Autodesk Fusion 360 part; units mm, degrees
(part 3 of 5)
sketch "草图7 (11)" plane through (0, 0, 0) normal (0, 0, 1) x (1, 0, 0) in component "RS_Integrated"
  line L0 (779, 145) -> (860, 145)
  line L1 (860, 145) -> (860, 153)
  line L2 (860, 153) -> (779, 153)
  line L3 (779, 153) -> (779, 145)
  dimension "d1107" = 779
  dimension "d1108" = 145
  dimension "d1109" = 81
  dimension "d1110" = 8
  constraint horizontal L0
  constraint vertical L1
  constraint horizontal L2
  constraint vertical L3
  measures "d1107" horizontal distance of origin L0.start
  measures "d1108" vertical distance of origin L0.start
  measures "d1109" horizontal distance of L0.start L0.end
  measures "d1110" vertical distance of L0.end L1.end
extrude "R05 low integral runner 0'''''" add sketch "草图7 (11)" along normal blind 10 bodies 11 in component "RS_Integrated"
ref_plane "工作平面8" through (0, 0, 0) normal (0, 0, 1) x (1, 0, 0) in component "RS_Integrated"
sketch "草图8 (11)" plane through (0, 0, 0) normal (0, 0, 1) x (1, 0, 0) in component "RS_Integrated"
  line L0 (779, 311) -> (860, 311)
  line L1 (860, 311) -> (860, 319)
  line L2 (860, 319) -> (779, 319)
  line L3 (779, 319) -> (779, 311)
  dimension "d1115" = 779
  dimension "d1116" = 311
  dimension "d1117" = 81
  dimension "d1118" = 8
  constraint horizontal L0
  constraint vertical L1
  constraint horizontal L2
  constraint vertical L3
  measures "d1115" horizontal distance of origin L0.start
  measures "d1116" vertical distance of origin L0.start
  measures "d1117" horizontal distance of L0.start L0.end
  measures "d1118" vertical distance of L0.end L1.end
extrude "R05 low integral runner 1'''''" add sketch "草图8 (11)" along normal blind 10 bodies 11 in component "RS_Integrated"
chamfer "倒角1''''''''''" distance 0.4 angle 45 5 edges at (813.5, 145, 35) (813.5, 319, 35) (857, 232, 35) (815, 142, 35) (815, 322, 35) on bodies 11 in component "RS_Integrated"
ref_plane "工作平面1" through (0, 0, 26) normal (0, 0, 1) x (1, 0, 0) in component "RS_RemovableGrate"
sketch "草图1 (12)" plane through (0, 0, 26) normal (0, 0, 1) x (1, 0, 0) in component "RS_RemovableGrate"
  line L0 (773.3, 145.3) -> (856.7, 145.3)
  line L1 (856.7, 145.3) -> (856.7, 318.7)
  line L2 (856.7, 318.7) -> (773.3, 318.7)
  line L3 (773.3, 318.7) -> (773.3, 145.3)
  dimension "d1124" = 773.3
  dimension "d1126" = 83.4
  dimension "d1127" = 173.4
  constraint horizontal L0
  constraint vertical L1
  constraint horizontal L2
  constraint vertical L3
  measures "d1124" horizontal distance of origin L0.start
  measures "d1126" horizontal distance of L0.start L0.end
  measures "d1127" vertical distance of L0.end L1.end
extrude "Horizontal removable deck'''''" add sketch "草图1 (12)" along normal blind 4 separate body makes body 12 in component "RS_RemovableGrate"
ref_plane "工作平面2" through (0, 0, 26) normal (0, 0, 1) x (1, 0, 0) in component "RS_RemovableGrate"
sketch "草图2 (12)" plane through (0, 0, 26) normal (0, 0, 1) x (1, 0, 0) in component "RS_RemovableGrate"
  line L0 (780.3, 160) -> (849.7, 160)
  line L1 (849.7, 160) -> (849.7, 164)
  line L2 (849.7, 164) -> (780.3, 164)
  line L3 (780.3, 164) -> (780.3, 160)
  dimension "d1132" = 780.3
  dimension "d1133" = 160
  dimension "d1134" = 69.4
  dimension "d1135" = 4
  constraint horizontal L0
  constraint vertical L1
  constraint horizontal L2
  constraint vertical L3
  measures "d1132" horizontal distance of origin L0.start
  measures "d1133" vertical distance of origin L0.start
  measures "d1134" horizontal distance of L0.start L0.end
  measures "d1135" vertical distance of L0.end L1.end
extrude "Drain slot 1'''''" cut sketch "草图2 (12)" along normal blind 4 bodies 12 in component "RS_RemovableGrate"
ref_plane "工作平面3" through (0, 0, 26) normal (0, 0, 1) x (1, 0, 0) in component "RS_RemovableGrate"
sketch "草图3 (12)" plane through (0, 0, 26) normal (0, 0, 1) x (1, 0, 0) in component "RS_RemovableGrate"
  line L0 (780.3, 170) -> (849.7, 170)
  line L1 (849.7, 170) -> (849.7, 174)
  line L2 (849.7, 174) -> (780.3, 174)
  line L3 (780.3, 174) -> (780.3, 170)
  dimension "d1140" = 780.3
  dimension "d1141" = 170
  dimension "d1142" = 69.4
  dimension "d1143" = 4
  constraint horizontal L0
  constraint vertical L1
  constraint horizontal L2
  constraint vertical L3
  measures "d1140" horizontal distance of origin L0.start
  measures "d1141" vertical distance of origin L0.start
  measures "d1142" horizontal distance of L0.start L0.end
  measures "d1143" vertical distance of L0.end L1.end
extrude "Drain slot 2'''''" cut sketch "草图3 (12)" along normal blind 4 bodies 12 in component "RS_RemovableGrate"
ref_plane "工作平面4" through (0, 0, 26) normal (0, 0, 1) x (1, 0, 0) in component "RS_RemovableGrate"
sketch "草图4 (12)" plane through (0, 0, 26) normal (0, 0, 1) x (1, 0, 0) in component "RS_RemovableGrate"
  line L0 (780.3, 180) -> (849.7, 180)
  line L1 (849.7, 180) -> (849.7, 184)
  line L2 (849.7, 184) -> (780.3, 184)
  line L3 (780.3, 184) -> (780.3, 180)
  dimension "d1148" = 780.3
  dimension "d1149" = 180
  dimension "d1150" = 69.4
  dimension "d1151" = 4
  constraint horizontal L0
  constraint vertical L1
  constraint horizontal L2
  constraint vertical L3
  measures "d1148" horizontal distance of origin L0.start
  measures "d1149" vertical distance of origin L0.start
  measures "d1150" horizontal distance of L0.start L0.end
  measures "d1151" vertical distance of L0.end L1.end
extrude "Drain slot 3'''''" cut sketch "草图4 (12)" along normal blind 4 bodies 12 in component "RS_RemovableGrate"
ref_plane "工作平面5" through (0, 0, 26) normal (0, 0, 1) x (1, 0, 0) in component "RS_RemovableGrate"
sketch "草图5 (12)" plane through (0, 0, 26) normal (0, 0, 1) x (1, 0, 0) in component "RS_RemovableGrate"
  line L0 (780.3, 190) -> (849.7, 190)
  line L1 (849.7, 190) -> (849.7, 194)
  line L2 (849.7, 194) -> (780.3, 194)
  line L3 (780.3, 194) -> (780.3, 190)
  dimension "d1156" = 780.3
  dimension "d1157" = 190
  dimension "d1158" = 69.4
  dimension "d1159" = 4
  constraint horizontal L0
  constraint vertical L1
  constraint horizontal L2
  constraint vertical L3
  measures "d1156" horizontal distance of origin L0.start
  measures "d1157" vertical distance of origin L0.start
  measures "d1158" horizontal distance of L0.start L0.end
  measures "d1159" vertical distance of L0.end L1.end
extrude "Drain slot 4'''''" cut sketch "草图5 (12)" along normal blind 4 bodies 12 in component "RS_RemovableGrate"
ref_plane "工作平面6" through (0, 0, 26) normal (0, 0, 1) x (1, 0, 0) in component "RS_RemovableGrate"
sketch "草图6 (12)" plane through (0, 0, 26) normal (0, 0, 1) x (1, 0, 0) in component "RS_RemovableGrate"
  line L0 (780.3, 200) -> (849.7, 200)
  line L1 (849.7, 200) -> (849.7, 204)
  line L2 (849.7, 204) -> (780.3, 204)
  line L3 (780.3, 204) -> (780.3, 200)
  dimension "d1164" = 780.3
  dimension "d1165" = 200
  dimension "d1166" = 69.4
  dimension "d1167" = 4
  constraint horizontal L0
  constraint vertical L1
  constraint horizontal L2
  constraint vertical L3
  measures "d1164" horizontal distance of origin L0.start
  measures "d1165" vertical distance of origin L0.start
  measures "d1166" horizontal distance of L0.start L0.end
  measures "d1167" vertical distance of L0.end L1.end
extrude "Drain slot 5'''''" cut sketch "草图6 (12)" along normal blind 4 bodies 12 in component "RS_RemovableGrate"
ref_plane "工作平面7" through (0, 0, 26) normal (0, 0, 1) x (1, 0, 0) in component "RS_RemovableGrate"
sketch "草图7 (12)" plane through (0, 0, 26) normal (0, 0, 1) x (1, 0, 0) in component "RS_RemovableGrate"
  line L0 (780.3, 210) -> (849.7, 210)
  line L1 (849.7, 210) -> (849.7, 214)
  line L2 (849.7, 214) -> (780.3, 214)
  line L3 (780.3, 214) -> (780.3, 210)
  dimension "d1172" = 780.3
  dimension "d1173" = 210
  dimension "d1174" = 69.4
  dimension "d1175" = 4
  constraint horizontal L0
  constraint vertical L1
  constraint horizontal L2
  constraint vertical L3
  measures "d1172" horizontal distance of origin L0.start
  measures "d1173" vertical distance of origin L0.start
  measures "d1174" horizontal distance of L0.start L0.end
  measures "d1175" vertical distance of L0.end L1.end
extrude "Drain slot 6'''''" cut sketch "草图7 (12)" along normal blind 4 bodies 12 in component "RS_RemovableGrate"
ref_plane "工作平面8" through (0, 0, 26) normal (0, 0, 1) x (1, 0, 0) in component "RS_RemovableGrate"
sketch "草图8 (12)" plane through (0, 0, 26) normal (0, 0, 1) x (1, 0, 0) in component "RS_RemovableGrate"
  line L0 (780.3, 220) -> (849.7, 220)
  line L1 (849.7, 220) -> (849.7, 224)
  line L2 (849.7, 224) -> (780.3, 224)
  line L3 (780.3, 224) -> (780.3, 220)
  dimension "d1180" = 780.3
  dimension "d1181" = 220
  dimension "d1182" = 69.4
  dimension "d1183" = 4
  constraint horizontal L0
  constraint vertical L1
  constraint horizontal L2
  constraint vertical L3
  measures "d1180" horizontal distance of origin L0.start
  measures "d1181" vertical distance of origin L0.start
  measures "d1182" horizontal distance of L0.start L0.end
  measures "d1183" vertical distance of L0.end L1.end
extrude "Drain slot 7'''''" cut sketch "草图8 (12)" along normal blind 4 bodies 12 in component "RS_RemovableGrate"
ref_plane "工作平面9" through (0, 0, 26) normal (0, 0, 1) x (1, 0, 0) in component "RS_RemovableGrate"
sketch "草图9 (6)" plane through (0, 0, 26) normal (0, 0, 1) x (1, 0, 0) in component "RS_RemovableGrate"
  line L0 (780.3, 230) -> (849.7, 230)
  line L1 (849.7, 230) -> (849.7, 234)
  line L2 (849.7, 234) -> (780.3, 234)
  line L3 (780.3, 234) -> (780.3, 230)
  dimension "d1188" = 780.3
  dimension "d1189" = 230
  dimension "d1190" = 69.4
  dimension "d1191" = 4
  constraint horizontal L0
  constraint vertical L1
  constraint horizontal L2
  constraint vertical L3
  measures "d1188" horizontal distance of origin L0.start
  measures "d1189" vertical distance of origin L0.start
  measures "d1190" horizontal distance of L0.start L0.end
  measures "d1191" vertical distance of L0.end L1.end
extrude "Drain slot 8'''''" cut sketch "草图9 (6)" along normal blind 4 bodies 12 in component "RS_RemovableGrate"
ref_plane "工作平面10" through (0, 0, 26) normal (0, 0, 1) x (1, 0, 0) in component "RS_RemovableGrate"
sketch "草图10 (6)" plane through (0, 0, 26) normal (0, 0, 1) x (1, 0, 0) in component "RS_RemovableGrate"
  line L0 (780.3, 240) -> (849.7, 240)
  line L1 (849.7, 240) -> (849.7, 244)
  line L2 (849.7, 244) -> (780.3, 244)
  line L3 (780.3, 244) -> (780.3, 240)
  dimension "d1196" = 780.3
  dimension "d1197" = 240
  dimension "d1198" = 69.4
  dimension "d1199" = 4
  constraint horizontal L0
  constraint vertical L1
  constraint horizontal L2
  constraint vertical L3
  measures "d1196" horizontal distance of origin L0.start
  measures "d1197" vertical distance of origin L0.start
  measures "d1198" horizontal distance of L0.start L0.end
  measures "d1199" vertical distance of L0.end L1.end
extrude "Drain slot 9'''''" cut sketch "草图10 (6)" along normal blind 4 bodies 12 in component "RS_RemovableGrate"
ref_plane "工作平面11" through (0, 0, 26) normal (0, 0, 1) x (1, 0, 0) in component "RS_RemovableGrate"
sketch "草图11 (6)" plane through (0, 0, 26) normal (0, 0, 1) x (1, 0, 0) in component "RS_RemovableGrate"
  line L0 (780.3, 250) -> (849.7, 250)
  line L1 (849.7, 250) -> (849.7, 254)
  line L2 (849.7, 254) -> (780.3, 254)
  line L3 (780.3, 254) -> (780.3, 250)
  dimension "d1204" = 780.3
  dimension "d1205" = 250
  dimension "d1206" = 69.4
  dimension "d1207" = 4
  constraint horizontal L0
  constraint vertical L1
  constraint horizontal L2
  constraint vertical L3
  measures "d1204" horizontal distance of origin L0.start
  measures "d1205" vertical distance of origin L0.start
  measures "d1206" horizontal distance of L0.start L0.end
  measures "d1207" vertical distance of L0.end L1.end
extrude "Drain slot 10'''''" cut sketch "草图11 (6)" along normal blind 4 bodies 12 in component "RS_RemovableGrate"
ref_plane "工作平面12" through (0, 0, 26) normal (0, 0, 1) x (1, 0, 0) in component "RS_RemovableGrate"
sketch "草图12 (6)" plane through (0, 0, 26) normal (0, 0, 1) x (1, 0, 0) in component "RS_RemovableGrate"
  line L0 (780.3, 260) -> (849.7, 260)
  line L1 (849.7, 260) -> (849.7, 264)
  line L2 (849.7, 264) -> (780.3, 264)
  line L3 (780.3, 264) -> (780.3, 260)
  dimension "d1212" = 780.3
  dimension "d1213" = 260
  dimension "d1214" = 69.4
  dimension "d1215" = 4
  constraint horizontal L0
  constraint vertical L1
  constraint horizontal L2
  constraint vertical L3
  measures "d1212" horizontal distance of origin L0.start
  measures "d1213" vertical distance of origin L0.start
  measures "d1214" horizontal distance of L0.start L0.end
  measures "d1215" vertical distance of L0.end L1.end
extrude "Drain slot 11'''''" cut sketch "草图12 (6)" along normal blind 4 bodies 12 in component "RS_RemovableGrate"
ref_plane "工作平面13" through (0, 0, 26) normal (0, 0, 1) x (1, 0, 0) in component "RS_RemovableGrate"
sketch "草图13 (4)" plane through (0, 0, 26) normal (0, 0, 1) x (1, 0, 0) in component "RS_RemovableGrate"
  line L0 (780.3, 270) -> (849.7, 270)
  line L1 (849.7, 270) -> (849.7, 274)
  line L2 (849.7, 274) -> (780.3, 274)
  line L3 (780.3, 274) -> (780.3, 270)
  dimension "d1220" = 780.3
  dimension "d1221" = 270
  dimension "d1222" = 69.4
  dimension "d1223" = 4
  constraint horizontal L0
  constraint vertical L1
  constraint horizontal L2
  constraint vertical L3
  measures "d1220" horizontal distance of origin L0.start
  measures "d1221" vertical distance of origin L0.start
  measures "d1222" horizontal distance of L0.start L0.end
  measures "d1223" vertical distance of L0.end L1.end
extrude "Drain slot 12'''" cut sketch "草图13 (4)" along normal blind 4 bodies 12 in component "RS_RemovableGrate"
ref_plane "工作平面14" through (0, 0, 26) normal (0, 0, 1) x (1, 0, 0) in component "RS_RemovableGrate"
sketch "草图14 (4)" plane through (0, 0, 26) normal (0, 0, 1) x (1, 0, 0) in component "RS_RemovableGrate"
  line L0 (780.3, 280) -> (849.7, 280)
  line L1 (849.7, 280) -> (849.7, 284)
  line L2 (849.7, 284) -> (780.3, 284)
  line L3 (780.3, 284) -> (780.3, 280)
  dimension "d1228" = 780.3
  dimension "d1229" = 280
  dimension "d1230" = 69.4
  dimension "d1231" = 4
  constraint horizontal L0
  constraint vertical L1
  constraint horizontal L2
  constraint vertical L3
  measures "d1228" horizontal distance of origin L0.start
  measures "d1229" vertical distance of origin L0.start
  measures "d1230" horizontal distance of L0.start L0.end
  measures "d1231" vertical distance of L0.end L1.end
extrude "Drain slot 13'''" cut sketch "草图14 (4)" along normal blind 4 bodies 12 in component "RS_RemovableGrate"
ref_plane "工作平面15" through (0, 0, 26) normal (0, 0, 1) x (1, 0, 0) in component "RS_RemovableGrate"
sketch "草图15 (4)" plane through (0, 0, 26) normal (0, 0, 1) x (1, 0, 0) in component "RS_RemovableGrate"
  line L0 (780.3, 290) -> (849.7, 290)
  line L1 (849.7, 290) -> (849.7, 294)
  line L2 (849.7, 294) -> (780.3, 294)
  line L3 (780.3, 294) -> (780.3, 290)
  dimension "d1236" = 780.3
  dimension "d1237" = 290
  dimension "d1238" = 69.4
  dimension "d1239" = 4
  constraint horizontal L0
  constraint vertical L1
  constraint horizontal L2
  constraint vertical L3
  measures "d1236" horizontal distance of origin L0.start
  measures "d1237" vertical distance of origin L0.start
  measures "d1238" horizontal distance of L0.start L0.end
  measures "d1239" vertical distance of L0.end L1.end
extrude "Drain slot 14'''" cut sketch "草图15 (4)" along normal blind 4 bodies 12 in component "RS_RemovableGrate"
ref_plane "工作平面16" through (0, 0, 26) normal (0, 0, 1) x (1, 0, 0) in component "RS_RemovableGrate"
sketch "草图16 (4)" plane through (0, 0, 26) normal (0, 0, 1) x (1, 0, 0) in component "RS_RemovableGrate"
  line L0 (780.3, 300) -> (849.7, 300)
  line L1 (849.7, 300) -> (849.7, 304)
  line L2 (849.7, 304) -> (780.3, 304)
  line L3 (780.3, 304) -> (780.3, 300)
  dimension "d1244" = 780.3
  dimension "d1245" = 300
  dimension "d1246" = 69.4
  dimension "d1247" = 4
  constraint horizontal L0
  constraint vertical L1
  constraint horizontal L2
  constraint vertical L3
  measures "d1244" horizontal distance of origin L0.start
  measures "d1245" vertical distance of origin L0.start
  measures "d1246" horizontal distance of L0.start L0.end
  measures "d1247" vertical distance of L0.end L1.end
extrude "Drain slot 15'''" cut sketch "草图16 (4)" along normal blind 4 bodies 12 in component "RS_RemovableGrate"
chamfer "倒角1'''''''''''" distance 0.4 angle 45 4 edges at (815, 318.7, 30) (856.7, 232, 30) (815, 145.3, 30) (773.3, 232, 30) on bodies 12 in component "RS_RemovableGrate"
ref_plane "工作平面17" through (0, 0, 26) normal (0, 0, 1) x (1, 0, 0) in component "L1_RemovableGrate"
sketch "草图17 (2)" plane through (0, 0, 26) normal (0, 0, 1) x (1, 0, 0) in component "L1_RemovableGrate"
  line L0 (52.7, 59.7) -> (55.3, 59.7)
  line L1 (55.3, 59.7) -> (55.3, 65.3)
  line L2 (55.3, 65.3) -> (52.7, 65.3)
  line L3 (52.7, 65.3) -> (52.7, 59.7)
  dimension "d1254" = 59.7
  dimension "d1255" = 2.6
  dimension "d1256" = 5.6
  constraint horizontal L0
  constraint vertical L1
  constraint horizontal L2
  constraint vertical L3
  measures "d1254" vertical distance of origin L0.start
  measures "d1255" horizontal distance of L0.start L0.end
  measures "d1256" vertical distance of L0.end L1.end
extrude "R05 grate locating notch 0" cut sketch "草图17 (2)" along normal blind 4 bodies 4 in component "L1_RemovableGrate"
ref_plane "工作平面9" through (0, 0, 10) normal (0, 0, 1) x (1, 0, 0) in component "L1_Integrated"
sketch "草图9 (7)" plane through (0, 0, 10) normal (0, 0, 1) x (1, 0, 0) in component "L1_Integrated"
  line L0 (53, 60) -> (55, 60)
  line L1 (55, 60) -> (55, 65)
  line L2 (55, 65) -> (53, 65)
  line L3 (53, 65) -> (53, 60)
  dimension "d1262" = 60
  dimension "d1263" = 2
  dimension "d1264" = 5
  constraint horizontal L0
  constraint vertical L1
  constraint horizontal L2
  constraint vertical L3
  measures "d1262" vertical distance of origin L0.start
  measures "d1263" horizontal distance of L0.start L0.end
  measures "d1264" vertical distance of L0.end L1.end
extrude "R05 grate locating key 0" add sketch "草图9 (7)" along normal blind 20 bodies 3 in component "L1_Integrated"
ref_plane "工作平面18" through (0, 0, 26) normal (0, 0, 1) x (1, 0, 0) in component "L1_RemovableGrate"
sketch "草图18 (2)" plane through (0, 0, 26) normal (0, 0, 1) x (1, 0, 0) in component "L1_RemovableGrate"
  line L0 (224.7, 59.7) -> (227.3, 59.7)
  line L1 (227.3, 59.7) -> (227.3, 65.3)
  line L2 (227.3, 65.3) -> (224.7, 65.3)
  line L3 (224.7, 65.3) -> (224.7, 59.7)
  dimension "d1269" = 224.7
  dimension "d1270" = 59.7
  dimension "d1271" = 2.6
  dimension "d1272" = 5.6
  constraint horizontal L0
  constraint vertical L1
  constraint horizontal L2
  constraint vertical L3
  measures "d1269" horizontal distance of origin L0.start
  measures "d1270" vertical distance of origin L0.start
  measures "d1271" horizontal distance of L0.start L0.end
  measures "d1272" vertical distance of L0.end L1.end
extrude "R05 grate locating notch 1" cut sketch "草图18 (2)" along normal blind 4 bodies 4 in component "L1_RemovableGrate"
ref_plane "工作平面10" through (0, 0, 10) normal (0, 0, 1) x (1, 0, 0) in component "L1_Integrated"
sketch "草图10 (7)" plane through (0, 0, 10) normal (0, 0, 1) x (1, 0, 0) in component "L1_Integrated"
  line L0 (225, 60) -> (227, 60)
  line L1 (227, 60) -> (227, 65)
  line L2 (227, 65) -> (225, 65)
  line L3 (225, 65) -> (225, 60)
  dimension "d1277" = 225
  dimension "d1278" = 60
  dimension "d1279" = 2
  dimension "d1280" = 5
  constraint horizontal L0
  constraint vertical L1
  constraint horizontal L2
  constraint vertical L3
  measures "d1277" horizontal distance of origin L0.start
  measures "d1278" vertical distance of origin L0.start
  measures "d1279" horizontal distance of L0.start L0.end
  measures "d1280" vertical distance of L0.end L1.end
extrude "R05 grate locating key 1" add sketch "草图10 (7)" along normal blind 20 bodies 3 in component "L1_Integrated"
ref_plane "工作平面19" through (0, 0, 26) normal (0, 0, 1) x (1, 0, 0) in component "L2_RemovableGrate"
sketch "草图19" plane through (0, 0, 26) normal (0, 0, 1) x (1, 0, 0) in component "L2_RemovableGrate"
  line L0 (234.7, 59.7) -> (237.3, 59.7)
  line L1 (237.3, 59.7) -> (237.3, 65.3)
  line L2 (237.3, 65.3) -> (234.7, 65.3)
  line L3 (234.7, 65.3) -> (234.7, 59.7)
  dimension "d1286" = 59.7
  dimension "d1287" = 2.6
  dimension "d1288" = 5.6
  constraint horizontal L0
  constraint vertical L1
  constraint horizontal L2
  constraint vertical L3
  measures "d1286" vertical distance of origin L0.start
  measures "d1287" horizontal distance of L0.start L0.end
  measures "d1288" vertical distance of L0.end L1.end
extrude "R05 grate locating notch 0'" cut sketch "草图19" along normal blind 4 bodies 6 in component "L2_RemovableGrate"
ref_plane "工作平面9" through (0, 0, 10) normal (0, 0, 1) x (1, 0, 0) in component "L2_Integrated"
sketch "草图9 (8)" plane through (0, 0, 10) normal (0, 0, 1) x (1, 0, 0) in component "L2_Integrated"
  line L0 (235, 60) -> (237, 60)
  line L1 (237, 60) -> (237, 65)
  line L2 (237, 65) -> (235, 65)
  line L3 (235, 65) -> (235, 60)
  dimension "d1294" = 60
  dimension "d1295" = 2
  dimension "d1296" = 5
  constraint horizontal L0
  constraint vertical L1
  constraint horizontal L2
  constraint vertical L3
  measures "d1294" vertical distance of origin L0.start
  measures "d1295" horizontal distance of L0.start L0.end
  measures "d1296" vertical distance of L0.end L1.end
extrude "R05 grate locating key 0'" add sketch "草图9 (8)" along normal blind 20 bodies 5 in component "L2_Integrated"
ref_plane "工作平面20" through (0, 0, 26) normal (0, 0, 1) x (1, 0, 0) in component "L2_RemovableGrate"
sketch "草图20" plane through (0, 0, 26) normal (0, 0, 1) x (1, 0, 0) in component "L2_RemovableGrate"
  line L0 (424.7, 59.7) -> (427.3, 59.7)
  line L1 (427.3, 59.7) -> (427.3, 65.3)
  line L2 (427.3, 65.3) -> (424.7, 65.3)
  line L3 (424.7, 65.3) -> (424.7, 59.7)
  dimension "d1301" = 424.7
  dimension "d1302" = 59.7
  dimension "d1303" = 2.6
  dimension "d1304" = 5.6
  constraint horizontal L0
  constraint vertical L1
  constraint horizontal L2
  constraint vertical L3
  measures "d1301" horizontal distance of origin L0.start
  measures "d1302" vertical distance of origin L0.start
  measures "d1303" horizontal distance of L0.start L0.end
  measures "d1304" vertical distance of L0.end L1.end
extrude "R05 grate locating notch 1'" cut sketch "草图20" along normal blind 4 bodies 6 in component "L2_RemovableGrate"
ref_plane "工作平面10" through (0, 0, 10) normal (0, 0, 1) x (1, 0, 0) in component "L2_Integrated"
sketch "草图10 (8)" plane through (0, 0, 10) normal (0, 0, 1) x (1, 0, 0) in component "L2_Integrated"
  line L0 (425, 60) -> (427, 60)
  line L1 (427, 60) -> (427, 65)
  line L2 (427, 65) -> (425, 65)
  line L3 (425, 65) -> (425, 60)
  dimension "d1309" = 425
  dimension "d1310" = 60
  dimension "d1311" = 2
  dimension "d1312" = 5
  constraint horizontal L0
  constraint vertical L1
  constraint horizontal L2
  constraint vertical L3
  measures "d1309" horizontal distance of origin L0.start
  measures "d1310" vertical distance of origin L0.start
  measures "d1311" horizontal distance of L0.start L0.end
  measures "d1312" vertical distance of L0.end L1.end
extrude "R05 grate locating key 1'" add sketch "草图10 (8)" along normal blind 20 bodies 5 in component "L2_Integrated"
ref_plane "工作平面13" through (0, 0, 26) normal (0, 0, 1) x (1, 0, 0) in component "R1_RemovableGrate"
sketch "草图13 (5)" plane through (0, 0, 26) normal (0, 0, 1) x (1, 0, 0) in component "R1_RemovableGrate"
  line L0 (592.7, 59.7) -> (595.3, 59.7)
  line L1 (595.3, 59.7) -> (595.3, 65.3)
  line L2 (595.3, 65.3) -> (592.7, 65.3)
  line L3 (592.7, 65.3) -> (592.7, 59.7)
  dimension "d1318" = 59.7
  dimension "d1319" = 2.6
  dimension "d1320" = 5.6
  constraint horizontal L0
  constraint vertical L1
  constraint horizontal L2
  constraint vertical L3
  measures "d1318" vertical distance of origin L0.start
  measures "d1319" horizontal distance of L0.start L0.end
  measures "d1320" vertical distance of L0.end L1.end
extrude "R05 grate locating notch 0''" cut sketch "草图13 (5)" along normal blind 4 bodies 2 in component "R1_RemovableGrate"
ref_plane "工作平面9" through (0, 0, 10) normal (0, 0, 1) x (1, 0, 0) in component "R1_Integrated"
sketch "草图9 (9)" plane through (0, 0, 10) normal (0, 0, 1) x (1, 0, 0) in component "R1_Integrated"
  line L0 (593, 60) -> (595, 60)
  line L1 (595, 60) -> (595, 65)
  line L2 (595, 65) -> (593, 65)
  line L3 (593, 65) -> (593, 60)
  dimension "d1326" = 60
  dimension "d1327" = 2
  dimension "d1328" = 5
  constraint horizontal L0
  constraint vertical L1
  constraint horizontal L2
  constraint vertical L3
  measures "d1326" vertical distance of origin L0.start
  measures "d1327" horizontal distance of L0.start L0.end
  measures "d1328" vertical distance of L0.end L1.end
extrude "R05 grate locating key 0''" add sketch "草图9 (9)" along normal blind 20 bodies 1 in component "R1_Integrated"
ref_plane "工作平面14" through (0, 0, 26) normal (0, 0, 1) x (1, 0, 0) in component "R1_RemovableGrate"
sketch "草图14 (5)" plane through (0, 0, 26) normal (0, 0, 1) x (1, 0, 0) in component "R1_RemovableGrate"
  line L0 (718.7, 59.7) -> (721.3, 59.7)
  line L1 (721.3, 59.7) -> (721.3, 65.3)
  line L2 (721.3, 65.3) -> (718.7, 65.3)
  line L3 (718.7, 65.3) -> (718.7, 59.7)
  dimension "d1333" = 718.7
  dimension "d1334" = 59.7
  dimension "d1335" = 2.6
  dimension "d1336" = 5.6
  constraint horizontal L0
  constraint vertical L1
  constraint horizontal L2
  constraint vertical L3
  measures "d1333" horizontal distance of origin L0.start
  measures "d1334" vertical distance of origin L0.start
  measures "d1335" horizontal distance of L0.start L0.end
  measures "d1336" vertical distance of L0.end L1.end
extrude "R05 grate locating notch 1''" cut sketch "草图14 (5)" along normal blind 4 bodies 2 in component "R1_RemovableGrate"
ref_plane "工作平面10" through (0, 0, 10) normal (0, 0, 1) x (1, 0, 0) in component "R1_Integrated"
sketch "草图10 (9)" plane through (0, 0, 10) normal (0, 0, 1) x (1, 0, 0) in component "R1_Integrated"
  line L0 (719, 60) -> (721, 60)
  line L1 (721, 60) -> (721, 65)
  line L2 (721, 65) -> (719, 65)
  line L3 (719, 65) -> (719, 60)
  dimension "d1341" = 719
  dimension "d1342" = 60
  dimension "d1343" = 2
  dimension "d1344" = 5
  constraint horizontal L0
  constraint vertical L1
  constraint horizontal L2
  constraint vertical L3
  measures "d1341" horizontal distance of origin L0.start
  measures "d1342" vertical distance of origin L0.start
  measures "d1343" horizontal distance of L0.start L0.end
  measures "d1344" vertical distance of L0.end L1.end
extrude "R05 grate locating key 1''" add sketch "草图10 (9)" along normal blind 20 bodies 1 in component "R1_Integrated"
ref_plane "工作平面13" through (0, 0, 26) normal (0, 0, 1) x (1, 0, 0) in component "R2_RemovableGrate"
sketch "草图13 (6)" plane through (0, 0, 26) normal (0, 0, 1) x (1, 0, 0) in component "R2_RemovableGrate"
  line L0 (728.7, 59.7) -> (731.3, 59.7)
  line L1 (731.3, 59.7) -> (731.3, 65.3)
  line L2 (731.3, 65.3) -> (728.7, 65.3)
  line L3 (728.7, 65.3) -> (728.7, 59.7)
  dimension "d1349" = 728.7
  dimension "d1350" = 59.7
  dimension "d1351" = 2.6
  dimension "d1352" = 5.6
  constraint horizontal L0
  constraint vertical L1
  constraint horizontal L2
  constraint vertical L3
  measures "d1349" horizontal distance of origin L0.start
  measures "d1350" vertical distance of origin L0.start
  measures "d1351" horizontal distance of L0.start L0.end
  measures "d1352" vertical distance of L0.end L1.end
extrude "R05 grate locating notch 0'''" cut sketch "草图13 (6)" along normal blind 4 bodies 8 in component "R2_RemovableGrate"
ref_plane "工作平面9" through (0, 0, 10) normal (0, 0, 1) x (1, 0, 0) in component "R2_Integrated"
sketch "草图9 (10)" plane through (0, 0, 10) normal (0, 0, 1) x (1, 0, 0) in component "R2_Integrated"
  line L0 (729, 60) -> (731, 60)
  line L1 (731, 60) -> (731, 65)
  line L2 (731, 65) -> (729, 65)
  line L3 (729, 65) -> (729, 60)
  dimension "d1357" = 729
  dimension "d1358" = 60
  dimension "d1359" = 2
  dimension "d1360" = 5
  constraint horizontal L0
  constraint vertical L1
  constraint horizontal L2
  constraint vertical L3
  measures "d1357" horizontal distance of origin L0.start
  measures "d1358" vertical distance of origin L0.start
  measures "d1359" horizontal distance of L0.start L0.end
  measures "d1360" vertical distance of L0.end L1.end
extrude "R05 grate locating key 0'''" add sketch "草图9 (10)" along normal blind 20 bodies 7 in component "R2_Integrated"
ref_plane "工作平面14" through (0, 0, 26) normal (0, 0, 1) x (1, 0, 0) in component "R2_RemovableGrate"
sketch "草图14 (6)" plane through (0, 0, 26) normal (0, 0, 1) x (1, 0, 0) in component "R2_RemovableGrate"
  line L0 (854.7, 59.7) -> (857.3, 59.7)
  line L1 (857.3, 59.7) -> (857.3, 65.3)
  line L2 (857.3, 65.3) -> (854.7, 65.3)
  line L3 (854.7, 65.3) -> (854.7, 59.7)
  dimension "d1365" = 854.7
  dimension "d1366" = 59.7
  dimension "d1367" = 2.6
  dimension "d1368" = 5.6
  constraint horizontal L0
  constraint vertical L1
  constraint horizontal L2
  constraint vertical L3
  measures "d1365" horizontal distance of origin L0.start
  measures "d1366" vertical distance of origin L0.start
  measures "d1367" horizontal distance of L0.start L0.end
  measures "d1368" vertical distance of L0.end L1.end
extrude "R05 grate locating notch 1'''" cut sketch "草图14 (6)" along normal blind 4 bodies 8 in component "R2_RemovableGrate"
ref_plane "工作平面10" through (0, 0, 10) normal (0, 0, 1) x (1, 0, 0) in component "R2_Integrated"
sketch "草图10 (10)" plane through (0, 0, 10) normal (0, 0, 1) x (1, 0, 0) in component "R2_Integrated"
  line L0 (855, 60) -> (857, 60)
  line L1 (857, 60) -> (857, 65)
  line L2 (857, 65) -> (855, 65)
  line L3 (855, 65) -> (855, 60)
  dimension "d1373" = 855
  dimension "d1374" = 60
  dimension "d1375" = 2
  dimension "d1376" = 5
  constraint horizontal L0
  constraint vertical L1
  constraint horizontal L2
  constraint vertical L3
  measures "d1373" horizontal distance of origin L0.start
  measures "d1374" vertical distance of origin L0.start
  measures "d1375" horizontal distance of L0.start L0.end
  measures "d1376" vertical distance of L0.end L1.end
extrude "R05 grate locating key 1'''" add sketch "草图10 (10)" along normal blind 20 bodies 7 in component "R2_Integrated"
ref_plane "工作平面17" through (0, 0, 26) normal (0, 0, 1) x (1, 0, 0) in component "LS_RemovableGrate"
sketch "草图17 (3)" plane through (0, 0, 26) normal (0, 0, 1) x (1, 0, 0) in component "LS_RemovableGrate"
  line L0 (59.7, 316.7) -> (65.3, 316.7)
  line L1 (65.3, 316.7) -> (65.3, 319.3)
  line L2 (65.3, 319.3) -> (59.7, 319.3)
  line L3 (59.7, 319.3) -> (59.7, 316.7)
  dimension "d1381" = 59.7
  dimension "d1382" = 316.7
  dimension "d1383" = 5.6
  dimension "d1384" = 2.6
  constraint horizontal L0
  constraint vertical L1
  constraint horizontal L2
  constraint vertical L3
  measures "d1381" horizontal distance of origin L0.start
  measures "d1382" vertical distance of origin L0.start
  measures "d1383" horizontal distance of L0.start L0.end
  measures "d1384" vertical distance of L0.end L1.end
extrude "R05 grate locating notch 0''''" cut sketch "草图17 (3)" along normal blind 4 bodies 10 in component "LS_RemovableGrate"
ref_plane "工作平面9" through (0, 0, 10) normal (0, 0, 1) x (1, 0, 0) in component "LS_Integrated"
sketch "草图9 (11)" plane through (0, 0, 10) normal (0, 0, 1) x (1, 0, 0) in component "LS_Integrated"
  line L0 (60, 317) -> (65, 317)
  line L1 (65, 317) -> (65, 319)
  line L2 (65, 319) -> (60, 319)
  line L3 (60, 319) -> (60, 317)
  dimension "d1389" = 60
  dimension "d1390" = 317
  dimension "d1391" = 5
  dimension "d1392" = 2
  constraint horizontal L0
  constraint vertical L1
  constraint horizontal L2
  constraint vertical L3
  measures "d1389" horizontal distance of origin L0.start
  measures "d1390" vertical distance of origin L0.start
  measures "d1391" horizontal distance of L0.start L0.end
  measures "d1392" vertical distance of L0.end L1.end
extrude "R05 grate locating key 0''''" add sketch "草图9 (11)" along normal blind 20 bodies 9 in component "LS_Integrated"
ref_plane "工作平面18" through (0, 0, 26) normal (0, 0, 1) x (1, 0, 0) in component "LS_RemovableGrate"
sketch "草图18 (3)" plane through (0, 0, 26) normal (0, 0, 1) x (1, 0, 0) in component "LS_RemovableGrate"
  line L0 (59.7, 144.7) -> (65.3, 144.7)
  line L1 (65.3, 144.7) -> (65.3, 147.3)
  line L2 (65.3, 147.3) -> (59.7, 147.3)
  line L3 (59.7, 147.3) -> (59.7, 144.7)
  dimension "d1397" = 59.7
  dimension "d1398" = 144.7
  dimension "d1399" = 5.6
  dimension "d1400" = 2.6
  constraint horizontal L0
  constraint vertical L1
  constraint horizontal L2
  constraint vertical L3
  measures "d1397" horizontal distance of origin L0.start
  measures "d1398" vertical distance of origin L0.start
  measures "d1399" horizontal distance of L0.start L0.end
  measures "d1400" vertical distance of L0.end L1.end
extrude "R05 grate locating notch 1''''" cut sketch "草图18 (3)" along normal blind 4 bodies 10 in component "LS_RemovableGrate"
ref_plane "工作平面10" through (0, 0, 10) normal (0, 0, 1) x (1, 0, 0) in component "LS_Integrated"
sketch "草图10 (11)" plane through (0, 0, 10) normal (0, 0, 1) x (1, 0, 0) in component "LS_Integrated"
  line L0 (60, 145) -> (65, 145)
  line L1 (65, 145) -> (65, 147)
  line L2 (65, 147) -> (60, 147)
  line L3 (60, 147) -> (60, 145)
  dimension "d1405" = 60
  dimension "d1406" = 145
  dimension "d1407" = 5
  dimension "d1408" = 2
  constraint horizontal L0
  constraint vertical L1
  constraint horizontal L2
  constraint vertical L3
  measures "d1405" horizontal distance of origin L0.start
  measures "d1406" vertical distance of origin L0.start
  measures "d1407" horizontal distance of L0.start L0.end
  measures "d1408" vertical distance of L0.end L1.end
extrude "R05 grate locating key 1''''" add sketch "草图10 (11)" along normal blind 20 bodies 9 in component "LS_Integrated"
ref_plane "工作平面17" through (0, 0, 26) normal (0, 0, 1) x (1, 0, 0) in component "RS_RemovableGrate"
sketch "草图17 (4)" plane through (0, 0, 26) normal (0, 0, 1) x (1, 0, 0) in component "RS_RemovableGrate"
  line L0 (844.7, 144.7) -> (850.3, 144.7)
  line L1 (850.3, 144.7) -> (850.3, 147.3)
  line L2 (850.3, 147.3) -> (844.7, 147.3)
  line L3 (844.7, 147.3) -> (844.7, 144.7)
  dimension "d1413" = 844.7
  dimension "d1415" = 5.6
  dimension "d1416" = 2.6
  constraint horizontal L0
  constraint vertical L1
  constraint horizontal L2
  constraint vertical L3
  measures "d1413" horizontal distance of origin L0.start
  measures "d1415" horizontal distance of L0.start L0.end
  measures "d1416" vertical distance of L0.end L1.end
extrude "R05 grate locating notch 0'''''" cut sketch "草图17 (4)" along normal blind 4 bodies 12 in component "RS_RemovableGrate"
ref_plane "工作平面9" through (0, 0, 10) normal (0, 0, 1) x (1, 0, 0) in component "RS_Integrated"
sketch "草图9 (12)" plane through (0, 0, 10) normal (0, 0, 1) x (1, 0, 0) in component "RS_Integrated"
  line L0 (845, 145) -> (850, 145)
  line L1 (850, 145) -> (850, 147)
  line L2 (850, 147) -> (845, 147)
  line L3 (845, 147) -> (845, 145)
  dimension "d1421" = 845
  dimension "d1423" = 5
  dimension "d1424" = 2
  constraint horizontal L0
  constraint vertical L1
  constraint horizontal L2
  constraint vertical L3
  measures "d1421" horizontal distance of origin L0.start
  measures "d1423" horizontal distance of L0.start L0.end
  measures "d1424" vertical distance of L0.end L1.end
extrude "R05 grate locating key 0'''''" add sketch "草图9 (12)" along normal blind 20 bodies 11 in component "RS_Integrated"
ref_plane "工作平面18" through (0, 0, 26) normal (0, 0, 1) x (1, 0, 0) in component "RS_RemovableGrate"
sketch "草图18 (4)" plane through (0, 0, 26) normal (0, 0, 1) x (1, 0, 0) in component "RS_RemovableGrate"
  line L0 (844.7, 316.7) -> (850.3, 316.7)
  line L1 (850.3, 316.7) -> (850.3, 319.3)
  line L2 (850.3, 319.3) -> (844.7, 319.3)
  line L3 (844.7, 319.3) -> (844.7, 316.7)
  dimension "d1429" = 844.7
  dimension "d1430" = 316.7
  dimension "d1431" = 5.6
  dimension "d1432" = 2.6
  constraint horizontal L0
  constraint vertical L1
  constraint horizontal L2
  constraint vertical L3
  measures "d1429" horizontal distance of origin L0.start
  measures "d1430" vertical distance of origin L0.start
  measures "d1431" horizontal distance of L0.start L0.end
  measures "d1432" vertical distance of L0.end L1.end
extrude "R05 grate locating notch 1'''''" cut sketch "草图18 (4)" along normal blind 4 bodies 12 in component "RS_RemovableGrate"
ref_plane "工作平面10" through (0, 0, 10) normal (0, 0, 1) x (1, 0, 0) in component "RS_Integrated"
sketch "草图10 (12)" plane through (0, 0, 10) normal (0, 0, 1) x (1, 0, 0) in component "RS_Integrated"
  line L0 (845, 317) -> (850, 317)
  line L1 (850, 317) -> (850, 319)
  line L2 (850, 319) -> (845, 319)
  line L3 (845, 319) -> (845, 317)
  dimension "d1437" = 845
  dimension "d1438" = 317
  dimension "d1439" = 5
  dimension "d1440" = 2
  constraint horizontal L0
  constraint vertical L1
  constraint horizontal L2
  constraint vertical L3
  measures "d1437" horizontal distance of origin L0.start
  measures "d1438" vertical distance of origin L0.start
  measures "d1439" horizontal distance of L0.start L0.end
  measures "d1440" vertical distance of L0.end L1.end
extrude "R05 grate locating key 1'''''" add sketch "草图10 (12)" along normal blind 20 bodies 11 in component "RS_Integrated"
component "R1_Integrated" placed x (1, 0, 0) y (0, 1, 0) z (0, 0, 1) at (0, 0, 0)
component "R1_RemovableGrate" placed x (1, 0, 0) y (0, 1, 0) z (0, 0, 1) at (0, 0, 0)
component "L1_Integrated" placed x (1, 0, 0) y (0, 1, 0) z (0, 0, 1) at (0, 0, 0)
component "L1_RemovableGrate" placed x (1, 0, 0) y (0, 1, 0) z (0, 0, 1) at (0, 0, 0)
component "L2_Integrated" placed x (1, 0, 0) y (0, 1, 0) z (0, 0, 1) at (0, 0, 0)
component "L2_RemovableGrate" placed x (1, 0, 0) y (0, 1, 0) z (0, 0, 1) at (0, 0, 0)
component "R2_Integrated" placed x (1, 0, 0) y (0, 1, 0) z (0, 0, 1) at (0, 0, 0)
component "R2_RemovableGrate" placed x (1, 0, 0) y (0, 1, 0) z (0, 0, 1) at (0, 0, 0)
component "LS_Integrated" placed x (1, 0, 0) y (0, 1, 0) z (0, 0, 1) at (0, 0, 0)
component "LS_RemovableGrate" placed x (1, 0, 0) y (0, 1, 0) z (0, 0, 1) at (0, 0, 0)
component "RS_Integrated" placed x (1, 0, 0) y (0, 1, 0) z (0, 0, 1) at (0, 0, 0)
component "RS_RemovableGrate" placed x (1, 0, 0) y (0, 1, 0) z (0, 0, 1) at (0, 0, 0)
equation "LeftAvailable = 400 mm" comment "User approximate dimension: left of faucet"
equation "RightAvailable = 300 mm" comment "User approximate dimension: right of faucet"
equation "RearAvailable = 100 mm" comment "User approximate rear strip depth"
equation "LeftSideAvailable = 130 mm" comment "User approximate left strip width"
equation "MirrorClearance = 300 mm" comment "User approximate countertop to mirror cabinet"
equation "RightSideAvailable = 100 mm" comment "ASSUMPTION: awaiting measurement"
equation "LeftReach = 180 mm" comment "ASSUMPTION: forward side extension beyond rear rack"
equation "RightReach = 180 mm" comment "ASSUMPTION: forward side extension beyond rear rack"
equation "FaucetGap = 160 mm" comment "ASSUMPTION: faucet and lever clearance, awaiting measurement"
equation "LeftRun = LeftAvailable - 20 mm" comment "Design clearance allowance; check on site"
equation "RightRun = RightAvailable - 30 mm" comment "Design clearance allowance; check lever"
equation "Depth = RearAvailable - 10 mm" comment "Rear standing module depth"
equation "LeftSideDepth = LeftSideAvailable - 10 mm" comment "Left side module depth"
equation "RightSideDepth = RightSideAvailable - 10 mm" comment "Right side module depth, provisional"
equation "ModuleGap = 2 mm" comment "Open cleaning / assembly seam, not watertight"
equation "TowerWidth = 180 mm" comment "Local upper tier only"
equation "TowerFrame = 8 mm" comment "Side portal frame thickness"
equation "TowerClearance = 2 mm" comment "Clearance from lower tray to side frames"
equation "FootHeight = 10 mm" comment "Clear gap below pan"
equation "PanHeight = 20 mm" comment "Pan rim above underside"
equation "FloorMin = 3 mm" comment "Minimum pan floor at outlet"
equation "Wall = 3 mm" comment "Pan walls"
equation "DrainSlope = 6 deg" comment "Initial design slope; verify with water test"
equation "DeckThick = 4 mm" comment "Removable horizontal grate thickness"
equation "DeckClearance = 0.3 mm" comment "Per-side clearance; fit coupon required"
equation "RimBorder = 7 mm" comment "Solid grate border"
equation "SlotWidth = 4 mm" comment "Open slat gaps"
equation "SlotPitch = 10 mm" comment "Initial grate slot spacing"
equation "DrainWidth = 28 mm" comment "R01 construction history only: R02 opens the entire front between side walls"
equation "DrainExtension = 0 mm" comment "R05 no projection and no inherited thickness offset"
equation "UpperDeckHeight = 145 mm" comment "Small jars only; verify cabinet swing"
equation "FootSize = 16 mm" comment "Support foot footprint"
equation "PegSize = 8 mm" comment "Square locating peg"
equation "PegHeight = 1.5 mm" comment "Foot locating peg, not a locking fastener"
equation "FitClearance = 0.25 mm" comment "Per-side foot fit allowance; test first"
equation "BaseX = 50 mm" comment "Model datum offset"
equation "BaseY = 50 mm" comment "Model datum offset"
equation "FrontFootInset = 17 mm" comment "R02 front foot center inset; outer foot edge is 9 mm behind open lip"
equation "TouchChamfer = 0.4 mm" comment "R03 selected touch edges; excludes drainage lip and locator bearing faces"
equation "RunnerWidth = 8 mm" comment "R03 integral support rail thickness"
equation "RimLift = 5 mm" comment "Three retaining edges above horizontal grate"
equation "SeatReach = 7 mm" comment "Triangular seat projection from side wall"
equation "SeatLength = 24 mm" comment "Flow aligned triangular seat base"
equation "SeatTipRadius = 1 mm" comment "Rounded triangular flow tip"
equation "d45 = FootHeight"
equation "d47 = ( BaseX + LeftRun + FaucetGap ) + ( 0 mm )"
equation "d48 = ( BaseY ) + ( 0 mm )"
equation "d49 = ( RightRun - ModuleGap ) / 2"
equation "d50 = Depth"
equation "d51 = PanHeight + RimLift"
equation "d55 = ( BaseX + LeftRun + FaucetGap ) + ( Wall )"
equation "d57 = -( -( ( FootHeight ) + FloorMin + ( ( Depth ) - ( Wall ) ) * tan(DrainSlope) ) )"
equation "d58 = ( ( BaseY ) + ( Wall ) )"
equation "d59 = -( -( ( FootHeight ) + FloorMin + ( ( Depth ) - ( Depth ) ) * tan(DrainSlope) ) )"
equation "d60 = ( ( BaseY ) + ( Depth ) )"
equation "d61 = -( -( FootHeight + PanHeight + RimLift + 1 mm ) )"
equation "d62 = ( ( RightRun - ModuleGap ) / 2 ) - 2 * Wall"
equation "d64 = FootHeight"
equation "d66 = ( ( BaseX + LeftRun + FaucetGap ) + ( Wall ) )"
equation "d67 = ( ( BaseY ) + ( Wall ) )"
equation "d68 = ( ( BaseX + LeftRun + FaucetGap ) + ( Wall + SeatReach ) )"
equation "d69 = ( ( BaseY ) + ( ( Wall ) + SeatLength / 2 ) )"
equation "d70 = ( ( BaseY ) + ( ( Wall ) + SeatLength ) )"
equation "d71 = PanHeight - DeckThick"
equation "d74 = SeatTipRadius"
equation "d75 = FootHeight"
equation "d77 = ( ( BaseX + LeftRun + FaucetGap ) + ( Wall ) )"
equation "d78 = ( ( BaseY ) + ( ( Depth ) - Wall - SeatLength ) )"
equation "d79 = ( ( BaseX + LeftRun + FaucetGap ) + ( Wall + SeatReach ) )"
equation "d80 = ( ( BaseY ) + ( ( ( Depth ) - Wall - SeatLength ) + SeatLength / 2 ) )"
equation "d81 = ( ( BaseY ) + ( ( ( Depth ) - Wall - SeatLength ) + SeatLength ) )"
equation "d82 = PanHeight - DeckThick"
equation "d85 = SeatTipRadius"
equation "d86 = FootHeight"
equation "d88 = ( ( BaseX + LeftRun + FaucetGap ) + ( ( ( RightRun - ModuleGap ) / 2 ) - Wall ) )"
equation "d89 = ( ( BaseY ) + ( Wall ) )"
equation "d90 = ( ( BaseX + LeftRun + FaucetGap ) + ( ( ( RightRun - ModuleGap ) / 2 ) - Wall - SeatReach ) )"
equation "d91 = ( ( BaseY ) + ( ( Wall ) + SeatLength / 2 ) )"
equation "d92 = ( ( BaseY ) + ( ( Wall ) + SeatLength ) )"
equation "d93 = PanHeight - DeckThick"
equation "d96 = SeatTipRadius"
equation "d97 = FootHeight"
equation "d99 = ( ( BaseX + LeftRun + FaucetGap ) + ( ( ( RightRun - ModuleGap ) / 2 ) - Wall ) )"
equation "d100 = ( ( BaseY ) + ( ( Depth ) - Wall - SeatLength ) )"
equation "d101 = ( ( BaseX + LeftRun + FaucetGap ) + ( ( ( RightRun - ModuleGap ) / 2 ) - Wall - SeatReach ) )"
equation "d102 = ( ( BaseY ) + ( ( ( Depth ) - Wall - SeatLength ) + SeatLength / 2 ) )"
equation "d103 = ( ( BaseY ) + ( ( ( Depth ) - Wall - SeatLength ) + SeatLength ) )"
equation "d104 = PanHeight - DeckThick"
equation "d107 = SeatTipRadius"
equation "d110 = ( BaseX + LeftRun + FaucetGap ) + ( 3 mm )"
equation "d111 = ( BaseY ) + ( 0 mm )"
equation "d112 = RunnerWidth"
equation "d113 = ( Depth ) - 9 mm"
equation "d114 = FootHeight"
equation "d118 = ( BaseX + LeftRun + FaucetGap ) + ( ( ( RightRun - ModuleGap ) / 2 ) - 3 mm - RunnerWidth )"
equation "d119 = ( BaseY ) + ( 0 mm )"
equation "d120 = RunnerWidth"
equation "d121 = ( Depth ) - 9 mm"
equation "d122 = FootHeight"
equation "d124 = TouchChamfer"
equation "d125 = ( FootHeight ) + PanHeight - DeckThick"
equation "d127 = ( BaseX + LeftRun + FaucetGap ) + ( Wall + DeckClearance )"
equation "d128 = ( BaseY ) + ( Wall + DeckClearance )"
equation "d129 = ( ( RightRun - ModuleGap ) / 2 ) - 2 * ( Wall + DeckClearance )"
equation "d130 = ( Depth ) - 2 * ( Wall + DeckClearance )"
equation "d131 = DeckThick"
equation "d133 = ( FootHeight ) + PanHeight - DeckThick"
equation "d135 = ( BaseX + LeftRun + FaucetGap ) + ( ( ( ( ( RightRun - ModuleGap ) / 2 ) - ( 10 * SlotPitch + SlotWidth ) ) / 2 ) + ( 0 * SlotPitch ) )"
equation "d136 = ( BaseY ) + ( Wall + DeckClearance + RimBorder )"
equation "d137 = SlotWidth"
equation "d138 = ( Depth ) - 2 * ( Wall + DeckClearance + RimBorder )"
equation "d139 = DeckThick"
equation "d141 = ( FootHeight ) + PanHeight - DeckThick"
equation "d143 = ( BaseX + LeftRun + FaucetGap ) + ( ( ( ( ( RightRun - ModuleGap ) / 2 ) - ( 10 * SlotPitch + SlotWidth ) ) / 2 ) + ( 1 * SlotPitch ) )"
equation "d144 = ( BaseY ) + ( Wall + DeckClearance + RimBorder )"
equation "d145 = SlotWidth"
equation "d146 = ( Depth ) - 2 * ( Wall + DeckClearance + RimBorder )"
equation "d147 = DeckThick"
equation "d149 = ( FootHeight ) + PanHeight - DeckThick"
equation "d151 = ( BaseX + LeftRun + FaucetGap ) + ( ( ( ( ( RightRun - ModuleGap ) / 2 ) - ( 10 * SlotPitch + SlotWidth ) ) / 2 ) + ( 2 * SlotPitch ) )"
equation "d152 = ( BaseY ) + ( Wall + DeckClearance + RimBorder )"
equation "d153 = SlotWidth"
equation "d154 = ( Depth ) - 2 * ( Wall + DeckClearance + RimBorder )"
equation "d155 = DeckThick"
equation "d157 = ( FootHeight ) + PanHeight - DeckThick"
equation "d159 = ( BaseX + LeftRun + FaucetGap ) + ( ( ( ( ( RightRun - ModuleGap ) / 2 ) - ( 10 * SlotPitch + SlotWidth ) ) / 2 ) + ( 3 * SlotPitch ) )"
equation "d160 = ( BaseY ) + ( Wall + DeckClearance + RimBorder )"
equation "d161 = SlotWidth"
equation "d162 = ( Depth ) - 2 * ( Wall + DeckClearance + RimBorder )"
equation "d163 = DeckThick"
equation "d165 = ( FootHeight ) + PanHeight - DeckThick"
equation "d167 = ( BaseX + LeftRun + FaucetGap ) + ( ( ( ( ( RightRun - ModuleGap ) / 2 ) - ( 10 * SlotPitch + SlotWidth ) ) / 2 ) + ( 4 * SlotPitch ) )"
equation "d168 = ( BaseY ) + ( Wall + DeckClearance + RimBorder )"
equation "d169 = SlotWidth"
equation "d170 = ( Depth ) - 2 * ( Wall + DeckClearance + RimBorder )"
equation "d171 = DeckThick"
equation "d173 = ( FootHeight ) + PanHeight - DeckThick"
equation "d175 = ( BaseX + LeftRun + FaucetGap ) + ( ( ( ( ( RightRun - ModuleGap ) / 2 ) - ( 10 * SlotPitch + SlotWidth ) ) / 2 ) + ( 5 * SlotPitch ) )"
equation "d176 = ( BaseY ) + ( Wall + DeckClearance + RimBorder )"
equation "d177 = SlotWidth"
equation "d178 = ( Depth ) - 2 * ( Wall + DeckClearance + RimBorder )"
equation "d179 = DeckThick"
equation "d181 = ( FootHeight ) + PanHeight - DeckThick"
equation "d183 = ( BaseX + LeftRun + FaucetGap ) + ( ( ( ( ( RightRun - ModuleGap ) / 2 ) - ( 10 * SlotPitch + SlotWidth ) ) / 2 ) + ( 6 * SlotPitch ) )"
equation "d184 = ( BaseY ) + ( Wall + DeckClearance + RimBorder )"
equation "d185 = SlotWidth"
equation "d186 = ( Depth ) - 2 * ( Wall + DeckClearance + RimBorder )"
equation "d187 = DeckThick"
equation "d189 = ( FootHeight ) + PanHeight - DeckThick"
equation "d191 = ( BaseX + LeftRun + FaucetGap ) + ( ( ( ( ( RightRun - ModuleGap ) / 2 ) - ( 10 * SlotPitch + SlotWidth ) ) / 2 ) + ( 7 * SlotPitch ) )"
equation "d192 = ( BaseY ) + ( Wall + DeckClearance + RimBorder )"
equation "d193 = SlotWidth"
equation "d194 = ( Depth ) - 2 * ( Wall + DeckClearance + RimBorder )"
equation "d195 = DeckThick"
equation "d197 = ( FootHeight ) + PanHeight - DeckThick"
equation "d199 = ( BaseX + LeftRun + FaucetGap ) + ( ( ( ( ( RightRun - ModuleGap ) / 2 ) - ( 10 * SlotPitch + SlotWidth ) ) / 2 ) + ( 8 * SlotPitch ) )"
equation "d200 = ( BaseY ) + ( Wall + DeckClearance + RimBorder )"
equation "d201 = SlotWidth"
equation "d202 = ( Depth ) - 2 * ( Wall + DeckClearance + RimBorder )"
equation "d203 = DeckThick"
equation "d205 = ( FootHeight ) + PanHeight - DeckThick"
equation "d207 = ( BaseX + LeftRun + FaucetGap ) + ( ( ( ( ( RightRun - ModuleGap ) / 2 ) - ( 10 * SlotPitch + SlotWidth ) ) / 2 ) + ( 9 * SlotPitch ) )"
equation "d208 = ( BaseY ) + ( Wall + DeckClearance + RimBorder )"
equation "d209 = SlotWidth"
equation "d210 = ( Depth ) - 2 * ( Wall + DeckClearance + RimBorder )"
equation "d211 = DeckThick"
equation "d213 = ( FootHeight ) + PanHeight - DeckThick"
equation "d215 = ( BaseX + LeftRun + FaucetGap ) + ( ( ( ( ( RightRun - ModuleGap ) / 2 ) - ( 10 * SlotPitch + SlotWidth ) ) / 2 ) + ( 10 * SlotPitch ) )"
equation "d216 = ( BaseY ) + ( Wall + DeckClearance + RimBorder )"